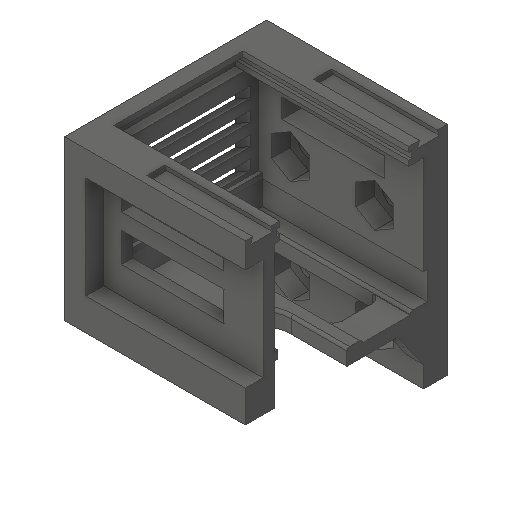
# Autodesk Inventor part: sensor-house-reflection
Saved by Autodesk Inventor 2022 (Build 260153000, 153)
## iProperties
Created: 2016-08-30
Part Number: sensor-house-reflection
Material: ABS Plastic
Document SubType Name: Modeling
Designer: Max
Density: 1.06 g/cm^3
Appearance: Gray
Mass: 12.7799 g
Surface Area: 104.372 cm^2
Volume: 12.0565 cm^3
Author: Max
Autodesk Inventor part; units mm, degrees
ref_plane "YZ Plane" through (0, 0, 0) normal (1, 0, 0) x (0, 1, 0)
ref_plane "XZ Plane" through (0, 0, 0) normal (0, 1, 0) x (-1, 0, 0)
ref_plane "XY Plane" through (0, 0, 0) normal (0, 0, 1) x (1, 0, 0)
sketch "Sketch1" plane through (0, 0, 0) normal (0, 1, 0) x (-1, 0, 0)
  line L0 (0, 0) -> (31.267, 0)
  line L1 (31.267, 0) -> (31.267, -29.05)
  line L2 (31.267, -29.05) -> (0, -29.05)
  line L3 (0, -29.05) -> (0, 0)
  line L4 (34.267, -32.05) -> (34.267, 3)
  line L5 (34.267, 3) -> (-3, 3)
  line L6 (-3, 3) -> (-3, -32.05)
  line L7 (-3, -32.05) -> (34.267, -32.05)
  line L8 (0, 3) -> (0, 0)
  line L9 (0, -29.05) -> (0, -32.05)
  dimension "d0" = 29.05
  dimension "d1" = 31.267
  dimension "d2" = 3
  constraints: 20 end point, 4 parallel, 3 point on line, 2 perpendicular, 1 horizontal, 1 vertical, 3 other
  measures "d0" distance of L0.end L1.end
  measures "d1" distance of L1.end L2.end
  measures "d2" distance between parallel lines of L1 L4
extrude "Extrusion1" add sketch "Sketch1" along normal blind 6.26 contours L8 L5 L4 L7 L9 L2 L1 L0
sketch "Sketch2" plane through (0, 6.26, 0) normal (0, 1, 0) x (1, 0, 0)
  line L0 (0, 0) -> (-31.267, 0) construction
  line L1 (-31.267, 0) -> (-31.267, 29.05) construction
  line L2 (-31.267, 29.05) -> (0, 29.05) construction
  line L3 (0, 29.05) -> (0, 32.05) construction
  line L4 (0, 32.05) -> (-34.267, 32.05) construction
  line L5 (-34.267, 32.05) -> (-34.267, -3) construction
  line L6 (-34.267, -3) -> (0, -3) construction
  line L7 (0, -3) -> (0, 0) construction
  line L8 (-34.267, 32.05) -> (-34.267, -3) projected
  line L9 (0, -3) -> (0, 0) projected
  line L10 (-34.267, -3) -> (0, -3)
  line L11 (0, -3) -> (0, 0.7)
  line L12 (0, 0.7) -> (-30.567, 0.7)
  line L13 (0, 0) -> (-31.267, 0) construction
  line L14 (-30.567, 0.7) -> (-30.567, 28.35)
  line L15 (-31.267, 0) -> (-31.267, 29.05) construction
  line L16 (-30.567, 28.35) -> (0, 28.35)
  line L17 (0, 29.05) -> (0, 32.05) projected
  line L18 (0, 28.35) -> (0, 32.05)
  line L19 (0, 32.05) -> (-34.267, 32.05) projected
  line L20 (0, 32.05) -> (-34.267, 32.05)
  line L21 (-34.267, 32.05) -> (-34.267, -3)
  dimension "d5" = 0.7
  dimension "d6" = 0.7
  dimension "d7" = 0.7
  constraints: 16 end point, 4 perpendicular, 2 parallel, 1 collinear, 1 horizontal, 1 point on line
  measures "d5" distance between parallel lines of L0 L12
  measures "d6" distance between parallel lines of L1 L14
  measures "d7" distance between parallel lines of L2 L16
extrude "Extrusion2" add sketch "Sketch2" against normal blind 1
sketch "Sketch3" plane through (0, 5.26, 0) normal (0, -1, 0) x (1, 0, 0)
  line L0 (-31.267, 0) -> (0, 0) construction
  line L1 (-31.267, -29.05) -> (-31.267, 0) construction
  line L2 (0, -29.05) -> (-31.267, -29.05) construction
  line L3 (0, -29.05) -> (0, -28.35) construction
  line L4 (0, -28.35) -> (-30.567, -28.35) construction
  line L5 (-30.567, -28.35) -> (-30.567, -0.7) construction
  line L6 (-30.567, -0.7) -> (0, -0.7) construction
  line L7 (0, -0.7) -> (0, 0) construction
  line L8 (0, -0.7) -> (0, 0) projected
  line L9 (0, 0) -> (-31.267, 0) projected
  line L10 (0, -0.7) -> (-30.567, -0.7)
  line L11 (-30.567, -0.7) -> (-30.567, 0)
  line L12 (-30.567, 0) -> (0, 0)
  line L13 (0, 0) -> (0, -0.7)
  constraints: 8 end point, 2 parallel, 1 collinear, 1 horizontal, 1 perpendicular, 1 point on line
extrude "Extrusion3" add sketch "Sketch3" along normal blind 0.5
sketch "Sketch4" plane through (0, 0, 0) normal (0, -1, 0) x (1, 0, 0)
  line L0 (0, 0) -> (-31.267, 0) projected
  line L1 (0, 3) -> (0, 0) projected
  line L2 (-34.267, 3) -> (0, 3) projected
  line L3 (-34.267, -32.05) -> (-34.267, 3) projected
  line L4 (0, -32.05) -> (-34.267, -32.05) projected
  line L5 (0, -29.05) -> (0, -32.05) projected
  line L6 (-31.267, -29.05) -> (0, -29.05) projected
  line L7 (-31.267, 0) -> (-31.267, -29.05) projected
extrude "Extrusion4" add sketch "Sketch4" against normal blind 24
sketch "Sketch7" plane through (0, 24, 0) normal (0, 1, 0) x (1, 0, 0)
  line L0 (0, 0.7) -> (-30.567, 0.7) construction
  line L1 (-30.567, 0.7) -> (-30.567, 28.35) construction
  line L2 (-30.567, 28.35) -> (0, 28.35) construction
  line L3 (-32.952, 1.015) -> (0, 1.015)
  line L4 (-32.952, 1.015) -> (-32.952, 25.535)
  line L5 (-32.952, 25.535) -> (0, 25.535)
  line L6 (0, -18.4949) -> (0, 56.6124) construction
  line L7 (-34.267, -3) -> (0, -3) projected
  line L8 (0, 1.015) -> (0, -3)
  line L9 (0, -3) -> (-34.267, -3)
  line L10 (-34.267, 32.05) -> (-34.267, -3) projected
  line L11 (-34.267, -3) -> (-34.267, 32.05)
  line L12 (-34.267, 32.05) -> (0, 32.05)
  line L13 (0, 29.05) -> (0, 32.05) projected
  line L14 (0, 25.535) -> (0, 32.05)
  point P0 (0, 0)
  dimension "d15" = 2.385
  dimension "d17" = 2.815
  dimension "d58" = 0.315
  constraints: 18 end point, 3 point on line, 3 vertical, 2 collinear, 2 horizontal, 2 perpendicular
  measures "d15" distance between parallel lines of L1 L4
  measures "d17" distance between parallel lines of L2 L5
  measures "d58" distance between parallel lines of L0 L3
extrude "Extrusion5" add sketch "Sketch7" along normal blind 1
sketch "Sketch8" plane through (0, 25, 0) normal (0, 1, 0) x (1, 0, 0)
  line L0 (0, 1.015) -> (-32.952, 1.015) construction
  line L1 (-32.952, 1.015) -> (-32.952, 25.535) construction
  line L2 (-32.952, 25.535) -> (0, 25.535) construction
  line L3 (0, 25.535) -> (0, 32.05) construction
  line L4 (0, 32.05) -> (-34.267, 32.05) construction
  line L5 (-34.267, 32.05) -> (-34.267, -3) construction
  line L6 (-34.267, -3) -> (0, -3) construction
  line L7 (0, -3) -> (0, 1.015) construction
  line L8 (0, -3) -> (0, 1.015) projected
  line L9 (0, 0.44) -> (-33.452, 0.44)
  line L10 (-33.452, 0.44) -> (-33.452, 26.11)
  line L11 (-33.452, 26.11) -> (0, 26.11)
  line L12 (0, 25.535) -> (0, 29.05) projected
  line L13 (0, 29.05) -> (0, 32.05) projected
  line L14 (0, 32.05) -> (-34.267, 32.05)
  line L15 (-34.267, -3) -> (0, -3) projected
  line L16 (-34.267, 32.05) -> (-34.267, -3) projected
  line L17 (-34.267, -3) -> (-34.267, 32.05)
  line L18 (-34.267, -3) -> (0, -3)
  line L19 (0, -3) -> (0, 0.44)
  line L20 (0, 26.11) -> (0, 32.05)
  point P0 (0, 0)
  dimension "d20" = 0.575
  dimension "d21" = 0.5
  dimension "d22" = 0.575
  constraints: 16 end point, 3 collinear, 3 perpendicular, 2 point on line, 1 horizontal, 1 vertical
  measures "d20" distance between parallel lines of L0 L9
  measures "d21" distance between parallel lines of L1 L10
  measures "d22" distance between parallel lines of L2 L11
extrude "Extrusion6" add sketch "Sketch8" along normal blind 1.25
sketch "Sketch9" plane through (0, 26.25, 0) normal (0, 1, 0) x (1, 0, 0)
  line L0 (0, 32.05) -> (-34.267, 32.05) construction
  line L1 (-34.267, 32.05) -> (-34.267, -3) construction
  line L2 (-34.267, -3) -> (0, -3) construction
  line L3 (0, -3) -> (0, 0.44) construction
  line L4 (0, 0.44) -> (-33.452, 0.44) construction
  line L5 (-33.452, 0.44) -> (-33.452, 26.11) construction
  line L6 (-33.452, 26.11) -> (0, 26.11) construction
  line L7 (0, 26.11) -> (0, 32.05) construction
  line L8 (0, 1.015) -> (-32.952, 1.015) construction
  line L9 (-32.952, 25.535) -> (0, 25.535) construction
  line L10 (-34.267, 32.05) -> (-34.267, -3) projected
  line L11 (-34.267, -3) -> (0, -3) projected
  line L12 (-34.267, -3) -> (0, -3)
  line L13 (-31.452, 1.015) -> (0, 1.015)
  line L14 (0, -3) -> (0, 1.015)
  line L15 (-31.452, 1.015) -> (-31.452, 25.535)
  line L16 (-31.452, 25.535) -> (0, 25.535)
  line L17 (0, 25.535) -> (0, 29.05) projected
  line L18 (0, 29.05) -> (0, 32.05) projected
  line L19 (0, 25.535) -> (0, 32.05)
  line L20 (0, 32.05) -> (-34.267, 32.05)
  line L21 (-34.267, -3) -> (-34.267, 32.05)
  dimension "d25" = 2
  constraints: 16 end point, 4 collinear, 2 perpendicular, 2 vertical, 1 point on line
  measures "d25" distance between parallel lines of L5 L15
extrude "Extrusion7" add sketch "Sketch9" along normal blind 1
sketch "Sketch10" plane through (0, 0, 0) normal (0, -1, 0) x (1, 0, 0)
  line L0 (-34.267, -32.05) -> (-34.267, 3) projected
  line L1 (0, -32.05) -> (-34.267, -32.05) projected
  line L2 (-34.267, 3) -> (0, 3)
  line L3 (0, 3) -> (0, -32.05)
  line L4 (0, -32.05) -> (-34.267, -32.05)
  line L5 (-34.267, -32.05) -> (-34.267, 3)
  point P0 (0, 0)
  constraints: 8 end point, 2 parallel, 1 horizontal, 1 perpendicular
extrude "Extrusion8" add sketch "Sketch10" along normal blind 3
sketch "Sketch11" plane through (0, -3, 0) normal (0, -1, 0) x (1, 0, 0)
  line L0 (-7.172, -16.735) -> (-26.102, -16.735)
  line L1 (-27.762, -18.395) -> (-27.762, -24.145)
  line L2 (-26.102, -25.805) -> (-7.172, -25.805)
  line L3 (-5.512, -24.145) -> (-5.512, -18.395)
  arc A0 (-5.512, -18.395) -> (-7.172, -16.735) centre (-7.172, -18.395) ccw
  arc A1 (-7.172, -25.805) -> (-5.512, -24.145) centre (-7.172, -24.145) ccw
  arc A2 (-26.102, -16.735) -> (-27.762, -18.395) centre (-26.102, -18.395) ccw
  arc A3 (-27.762, -24.145) -> (-26.102, -25.805) centre (-26.102, -24.145) ccw
  circle A4 centre (-10.572, -6.975) radius 6.835
  line L4 (-31.267, -29.05) -> (0, -29.05) construction
  line L5 (-31.267, 0) -> (-31.267, -29.05) construction
  line L6 (0, 0) -> (-31.267, 0) construction
  point P0 (-5.512, -16.735)
  point P1 (-27.762, -16.735)
  point P2 (-5.512, -25.805)
  dimension "d30" = 9.07
  dimension "d31" = 22.25
  dimension "d32" = 1.66
  dimension "d33" = 13.67
  dimension "d34" = 3.245
  dimension "d35" = 3.505
  dimension "d36" = 20.695
  dimension "d37" = 6.975
  constraints: 8 end point, 8 point on circle, 8 tangent, 6 point on line, 5 centre point, 3 equal radius, 2 parallel, 1 horizontal, 1 perpendicular
  measures "d30" distance of point (-5.512, -25.805) point (-5.512, -16.735)
  measures "d31" distance of point (-5.512, -16.735) point (-27.762, -16.735)
  measures "d32" radius of A0
  measures "d33" diameter of A4
  measures "d34" distance between parallel lines of L4 L2
  measures "d35" distance between parallel lines of L5 L1
  measures "d36" distance from line of L5 A4.centre
  measures "d37" distance from line of L6 A4.centre
extrude "Extrusion9" cut sketch "Sketch11" against normal blind 3
sketch "Sketch12" plane through (0, 24, -25.535) normal (1, 0, 0) x (0, 0, -1)
  line L0 (0.27, -27) -> (0.27, -24) construction
  line L1 (0.27, -27) -> (0.27, -24) construction
  line L2 (-8.8, -27) -> (-8.8, -24) construction
  line L3 (-8.8, -27) -> (-8.8, -24) construction
  line L4 (-8.8, -24) -> (0.27, -24)
  line L5 (0.27, -24) -> (0.27, -24.6)
  line L6 (0.27, -24.6) -> (-8.8, -24.6)
  line L7 (-8.8, -24.6) -> (-8.8, -24)
  point P0 (-25.535, -24)
  dimension "d40" = 0.6
  constraints: 8 end point, 2 parallel, 1 horizontal, 1 perpendicular, 1 point on line
  measures "d40" distance between parallel lines of L6 L4
extrude "Extrusion10" cut sketch "Sketch12" against normal blind 10
sketch "Sketch13" plane through (0, 24, -25.535) normal (1, 0, 0) x (0, 0, -1)
  line L0 (-25.395, -24) -> (-11.725, -24) construction
  line L1 (-11.725, -27) -> (-25.395, -27) construction
  line L2 (-25.395, -24) -> (-11.725, -24) projected
  line L3 (-25.395, -24) -> (-11.725, -24)
  line L4 (-11.725, -24) -> (-11.725, -27)
  line L5 (-11.725, -27) -> (-25.395, -27)
  line L6 (-25.395, -27) -> (-25.395, -24)
  point P0 (-25.535, -24)
  constraints: 8 end point, 2 parallel, 1 horizontal, 1 perpendicular
extrude "Extrusion11" cut sketch "Sketch13" against normal up to surface round surface about axis through (-10.572, -3, -6.975) along (0, 1, 0) radius 6.835 far side no
fillet "Fillet1" radius 0.5 8 edges at (-27.2758, 0, -17.2212) (-27.762, 0, -21.27) (-27.2758, 0, -25.3188) (-13.051, 0, -25.805) (-13.051, 0, -16.735) (-5.286, 0, -13.81) (-5.286, 0, -0.14) (-17.407, 0, -6.975)
sketch "Sketch16" plane through (-34.267, 27.25, 3) normal (0, 0, 1) x (1, 0, 0)
  line L0 (0, -30.25) -> (0, 0) construction
  line L1 (34.267, -30.25) -> (0, -30.25) construction
  line L2 (34.267, -30.25) -> (34.267, 0) construction
  line L3 (0, 0) -> (34.267, 0) construction
  line L4 (-13.0029, -10.46) -> (34.267, -10.46) construction
  line L5 (0, -7.185) -> (34.267, -7.185) construction
  line L6 (7.4, -6.758) -> (7.4, -10.36)
  line L7 (26.8405, -6.758) -> (26.8405, -10.46)
  line L8 (7.4, -6.758) -> (26.8405, -6.758)
  line L9 (7.4, -10.36) -> (26.8405, -10.36)
  point P0 (34.267, -27.25)
  dimension "d59" = 19.79
  dimension "d65" = 3.602
  dimension "d66" = 19.4405
  dimension "d67" = 7.4
  dimension "d155" = 10.36
  constraints: 12 end point, 5 point on line, 3 parallel, 2 horizontal, 1 vertical
  measures "d59" distance between parallel lines of L1 L4
  measures "d65" distance between parallel lines of L9 L8
  measures "d66" distance of L6.start L7.start
  measures "d67" distance between parallel lines of L0 L6
  measures "d155" distance between parallel lines of L3 L9
extrude "Extrusion14" cut sketch "Sketch16" against normal through all
thicken "Thicken1" operation add thickness 2.475 both sides no extend neighbours yes toward (0, 0, 1) faces at (-13.8978, 3.63, 3)
sketch "available_for_screw" plane through (-31.267, 6.26, -29.05) normal (0, 0, 1) x (1, 0, 0)
  line L0 (-0.185, 20.99) -> (31.267, 20.99) construction
  line L1 (1, 9.79) -> (30.267, 9.79) construction
  line L2 (30.267, 9.79) -> (30.267, 0.1) construction
  line L3 (30.267, 0.1) -> (1, 0.1) construction
  line L4 (1, 0.1) -> (1, 9.79) construction
  line L5 (31.267, 0) -> (0, 0) construction
  line L6 (0, 0) -> (0, 17.74) construction
  line L7 (31.267, 0) -> (31.267, 17.74) construction
  point P0 (31.267, -6.26)
  dimension "d82" = 11.2
  dimension "d83" = 0.1
  dimension "d84" = 1
  dimension "d85" = 1
  constraints: 8 end point, 2 parallel, 1 horizontal, 1 perpendicular
  measures "d82" distance between parallel lines of L1 L0
  measures "d83" distance between parallel lines of L5 L3
  measures "d84" distance between parallel lines of L6 L4
  measures "d85" distance between parallel lines of L7 L2
thicken "Thicken2" operation add thickness 0.8 both sides no extend neighbours yes toward (0, 0, -1) faces at (-13.8978, 3.63, -32.05)
sketch "Sketch20" plane through (-31.267, 6.26, -29.05) normal (0, 0, 1) x (1, 0, 0)
  line L0 (6, 1.1793) -> (2.44, 3.2346)
  line L1 (2.44, 3.2346) -> (2.44, 7.3454)
  line L2 (2.44, 7.3454) -> (6, 9.4007)
  line L3 (6, 9.4007) -> (9.56, 7.3454)
  line L4 (9.56, 7.3454) -> (9.56, 3.2346)
  line L5 (9.56, 3.2346) -> (6, 1.1793)
  line L6 (0, 0) -> (0, 17.74) projected
  line L7 (1, 9.79) -> (30.267, 9.79) construction
  circle A0 centre (6, 5.29) radius 2.04
  line L8 (22, 1.1793) -> (18.44, 3.2346)
  line L9 (18.44, 3.2346) -> (18.44, 7.3454)
  line L10 (18.44, 7.3454) -> (22, 9.4007)
  line L11 (22, 9.4007) -> (25.56, 7.3454)
  line L12 (25.56, 7.3454) -> (25.56, 3.2346)
  line L13 (25.56, 3.2346) -> (22, 1.1793)
  line L14 (31.267, 0) -> (31.267, 17.74) projected
  circle A1 centre (22, 5.29) radius 2.04
  point P0 (31.267, -6.26)
  dimension "d88" = 6
  dimension "d89" = 7.12
  dimension "d90" = 4.5
  dimension "d91" = 4.08
  dimension "d92" = 7.12
  dimension "d94" = 16
  dimension "d95" = 4.08
  constraints: 24 end point, 2 centre point, 2 coincident, 2 vertical, 1 horizontal alignment, 26 other
  measures "d88" distance from line of L6 point (6, 5.29)
  measures "d89" distance between parallel lines of L4 L1
  measures "d90" distance from line of point (6, 5.29) L7
  measures "d91" diameter of A0
  measures "d92" distance between parallel lines of L12 L9
  measures "d94" distance of point (6, 5.29) point (22, 5.29)
  measures "d95" diameter of A1
extrude "Extrusion17" cut sketch "Sketch20" against normal through all contours A0 | A1
extrude "Extrusion18" cut sketch "Sketch20" against normal blind 2.8
thicken "Thicken4" operation add thickness 0.7 both sides no extend neighbours yes toward (0, 0, 1) faces at (-12.8978, 22.8307, -29.05)
sketch "Sketch21" plane through (0, -3, -32.85) normal (0, 0, -1) x (-1, 0, 0)
  line L0 (34.267, 0) -> (0, 0) construction
  line L1 (0, 0) -> (34.267, 0)
  line L2 (34.267, 0) -> (34.267, -11)
  line L3 (34.267, -11) -> (0, -11)
  line L4 (0, -11) -> (0, 0)
  line L5 (34.267, 0) -> (34.267, 30.25) construction
  circle A0 centre (9.267, -5.1107) radius 2.04
  circle A1 centre (9.267, 14.55) radius 2.04 construction
  circle A2 centre (9.267, 14.55) radius 2.04 construction
  line L6 (9.267, 10.4393) -> (12.827, 12.4946) construction
  line L7 (5.707, 12.4946) -> (9.267, 10.4393) construction
  line L8 (5.707, 16.6054) -> (5.707, 12.4946) construction
  line L9 (9.267, 18.6607) -> (5.707, 16.6054) construction
  line L10 (12.827, 16.6054) -> (9.267, 18.6607) construction
  line L11 (12.827, 12.4946) -> (12.827, 16.6054) construction
  circle A3 centre (25.267, 14.55) radius 2.04 construction
  line L12 (25.267, 10.4393) -> (28.827, 12.4946) construction
  line L13 (21.707, 12.4946) -> (25.267, 10.4393) construction
  line L14 (21.707, 16.6054) -> (21.707, 12.4946) construction
  line L15 (25.267, 18.6607) -> (21.707, 16.6054) construction
  line L16 (28.827, 16.6054) -> (25.267, 18.6607) construction
  line L17 (28.827, 12.4946) -> (28.827, 16.6054) construction
  line L18 (9.267, -9.2215) -> (5.707, -7.1661)
  line L19 (5.707, -7.1661) -> (5.707, -3.0554)
  line L20 (5.707, -3.0554) -> (9.267, -1)
  line L21 (9.267, -1) -> (12.827, -3.0554)
  line L22 (12.827, -3.0554) -> (12.827, -7.1661)
  line L23 (12.827, -7.1661) -> (9.267, -9.2215)
  circle A4 centre (25.267, -5.1107) radius 2.04
  line L24 (25.267, -9.2215) -> (21.707, -7.1661)
  line L25 (21.707, -7.1661) -> (21.707, -3.0554)
  line L26 (21.707, -3.0554) -> (25.267, -1)
  line L27 (25.267, -1) -> (28.827, -3.0554)
  line L28 (28.827, -3.0554) -> (28.827, -7.1661)
  line L29 (28.827, -7.1661) -> (25.267, -9.2215)
  point P0 (0, 3)
  dimension "d104" = 11
  dimension "d105" = 7.12
  dimension "d106" = 1
  dimension "d107" = 4.08
  dimension "d108" = 4.08
  dimension "d109" = 7.12
  constraints: 32 end point, 2 centre point, 2 coincident, 2 parallel, 2 vertical, 2 vertical alignment, 1 collinear, 1 horizontal, 1 horizontal alignment, 1 perpendicular, 26 other
  measures "d104" distance of L3.end L0.end
  measures "d105" distance between parallel lines of L22 L19
  measures "d106" distance from line of L0 L20.end
  measures "d107" diameter of A0
  measures "d108" diameter of A4
  measures "d109" distance between parallel lines of L28 L25
extrude "Extrusion19" add sketch "Sketch21" against normal up to surface (4.5 mm away) contours L1 L2 L3 L4 | L18 L19 L20 L21 L22 L23 | L24 L25 L26 L27 L28 L29
sketch "Sketch22" plane through (-34.267, -3, -28.35) normal (0, 0, 1) x (1, 0, 0)
  line L0 (25, -1) -> (21.44, -3.0554) projected
  line L1 (28.56, -3.0554) -> (25, -1) projected
  line L2 (28.56, -7.1661) -> (28.56, -3.0554) projected
  line L3 (25, -9.2215) -> (28.56, -7.1661) projected
  line L4 (21.44, -7.1661) -> (25, -9.2215) projected
  line L5 (21.44, -3.0554) -> (21.44, -7.1661) projected
  line L6 (12.56, -7.1661) -> (12.56, -3.0554) projected
  line L7 (9, -9.2215) -> (12.56, -7.1661) projected
  line L8 (5.44, -7.1661) -> (9, -9.2215) projected
  line L9 (5.44, -3.0554) -> (5.44, -7.1661) projected
  line L10 (9, -1) -> (5.44, -3.0554) projected
  line L11 (12.56, -3.0554) -> (9, -1) projected
  point P0 (34.267, 3)
extrude "Extrusion20" cut sketch "Sketch22" against normal blind 3.5
sketch "Sketch24" plane through (-34.267, -3, 5.475) normal (-1, 0, 0) x (0, 0, 1)
  line L0 (-33.825, -11) -> (-33.825, 0) construction
  line L1 (0, 0) -> (-33.825, 0) construction
  line L2 (-33.825, -7.1661) -> (-33.825, -3.0554) construction
  line L3 (-33.825, -7) -> (-28.825, 0)
  line L4 (-33.825, -7) -> (-33.825, 0)
  line L5 (-28.825, 0) -> (-33.825, 0)
  point P0 (-5.475, 3)
  dimension "d118" = 5
  constraints: 6 end point, 1 collinear, 1 point on line, 1 vertical
  measures "d118" distance from line of L0 L3.end
extrude "Extrusion21" add sketch "Sketch24" against normal blind 3
sketch "Sketch25" plane through (0, 25, -26.11) normal (1, 0, 0) x (0, 0, -1)
  line L0 (-2.76, -28) -> (2.24, -35) projected
  line L1 (2.24, -28) -> (2.24, -35) projected
  line L2 (-2.76, -28) -> (2.24, -28) projected
  point P0 (-26.11, -25)
extrude "Extrusion22" add sketch "Sketch25" against normal blind 3
sketch "Sketch26" plane through (-34.267, -3, 5.475) normal (-1, 0, 0) x (0, 0, 1)
  line L0 (-32.325, 22.25) -> (-6, 22.25)
  line L1 (-6, 22.25) -> (-6, 20.25)
  line L2 (-6, 20.25) -> (-32.325, 20.25)
  line L3 (-32.325, 20.25) -> (-32.325, 22.25)
  line L4 (-33.825, -7) -> (-28.825, 0) construction
  line L5 (0, 0) -> (-28.825, 0) construction
  line L6 (0, 0) -> (0, 30.25) construction
  line L7 (-38.325, 30.25) -> (0, 30.25) construction
  line L8 (-38.325, -11) -> (-38.325, 30.25) construction
  line L9 (-33.825, 19.89) -> (-33.825, 23.492) construction
  line L10 (-33.825, 23.492) -> (-33.825, 19.89) construction
  line L11 (-33.825, 12.4946) -> (-33.825, 10.4393) construction
  line L12 (-33.825, 10.4393) -> (-33.825, 12.4946) construction
  line L13 (-33.825, 12.4946) -> (-33.825, 16.6054) construction
  line L14 (-33.825, 16.6054) -> (-33.825, 18.6607) construction
  line L15 (-33.825, 18.6607) -> (-33.825, 16.6054) construction
  line L16 (-33.825, 16.6054) -> (-33.825, 12.4946) construction
  line L17 (-33.825, 12.4946) -> (-33.825, 10.4393) construction
  line L18 (-33.825, 10.4393) -> (-33.825, 12.4946) construction
  line L19 (-33.825, 12.4946) -> (-33.825, 16.6054) construction
  line L20 (-33.825, 16.6054) -> (-33.825, 18.6607) construction
  line L21 (-33.825, 18.6607) -> (-33.825, 16.6054) construction
  line L22 (-33.825, 16.6054) -> (-33.825, 12.4946) construction
  line L23 (-33.825, 9.26) -> (-33.825, 8.26) construction
  line L24 (-33.825, 8.26) -> (-33.825, 27) construction
  line L25 (-33.825, 9.26) -> (-33.825, 27) construction
  line L26 (-32.325, 16.25) -> (-32.325, 18.25)
  line L27 (-6, 16.25) -> (-32.325, 16.25)
  line L28 (-32.325, 18.25) -> (-6, 18.25)
  line L29 (-6, 18.25) -> (-6, 16.25)
  line L30 (-32.325, 12.25) -> (-32.325, 14.25)
  line L31 (-6, 12.25) -> (-32.325, 12.25)
  line L32 (-32.325, 14.25) -> (-6, 14.25)
  line L33 (-6, 14.25) -> (-6, 12.25)
  line L34 (-32.325, 8.25) -> (-32.325, 10.25)
  line L35 (-6, 8.25) -> (-32.325, 8.25)
  line L36 (-32.325, 10.25) -> (-6, 10.25)
  line L37 (-6, 10.25) -> (-6, 8.25)
  line L38 (-38.325, -11) -> (-33.825, -11) projected
  line L39 (-33.825, -11) -> (-33.825, -7) projected
  point P0 (-5.475, 3)
  dimension "d124" = 8
  dimension "d125" = 2
  dimension "d126" = 6
  dimension "d127" = 6
  dimension "d130" = 4
  constraints: 32 end point, 2 parallel, 1 horizontal, 1 perpendicular, 1 vertical, 24 other
  measures "d124" distance between parallel lines of L7 L0
  measures "d125" distance of L2.end L0.start
  measures "d126" distance between parallel lines of L8 L3
  measures "d127" distance between parallel lines of L6 L1
  measures "d130" distance of L0.start L26.end
sketch "Sketch27" plane through (-34.267, -3, 5.475) normal (0, 0, 1) x (1, 0, 0)
  line L0 (34.267, 30.25) -> (0, 30.25) construction
  line L1 (0, 30.25) -> (4, 32.5594)
  point P0 (34.267, 3)
  dimension "d135" = 30
  dimension "d136" = 4
  constraints: 2 end point
  measures "d135" angle of L0 L1
  measures "d136" horizontal distance of L0.end L1.end
sweep "Sweep1" cut profiles "Sketch26" path "Sketch27"
sketch "Sketch28" plane through (-34.267, -3, 5.475) normal (0, 0, 1) x (1, 0, 0)
  line L0 (26.8405, 19.89) -> (7.4, 19.89) construction
  line L1 (7.4, 19.89) -> (7.4, 23.492) construction
  line L2 (7.4, 23.492) -> (26.8405, 23.492) construction
  line L3 (26.8405, 23.492) -> (26.8405, 19.89) construction
  line L4 (0, 0) -> (0, 30.25) construction
  line L5 (34.267, 0) -> (0, 0) construction
  line L6 (34.267, 0) -> (34.267, 30.25) construction
  line L7 (0, 30.25) -> (34.267, 30.25) construction
  line L8 (4, 25.492) -> (34.267, 25.492)
  line L9 (34.267, 25.492) -> (34.267, 6.0515)
  line L10 (34.267, 6.0515) -> (4, 6.0515)
  line L11 (4, 6.0515) -> (4, 25.492)
  line L12 (0, 0) -> (0, 30.25) construction
  point P0 (34.267, 3)
  dimension "d139" = 4
  dimension "d140" = 19.4405
  dimension "d141" = 2
  constraints: 8 end point, 2 parallel, 1 horizontal, 1 perpendicular, 1 point on line
  measures "d139" distance between parallel lines of L11 L12
  measures "d140" distance between parallel lines of L10 L8
  measures "d141" distance between parallel lines of L2 L8
extrude "Extrusion23" cut sketch "Sketch28" against normal blind 3.375
chamfer "Chamfer2" distance 4 angle 45 1 edges at (-34.267, -14, -30.6)
sketch "Sketch29" plane through (-34.267, -3, 2.1) normal (0, 0, 1) x (1, 0, 0)
  line L0 (26.8405, 23.492) -> (7.4, 23.492) construction
  line L1 (26.8405, 19.89) -> (26.8405, 23.492) construction
  line L2 (7.4, 19.89) -> (26.8405, 19.89) construction
  line L3 (7.4, 23.492) -> (7.4, 19.89) construction
  line L4 (4, 25.492) -> (34.267, 25.492) construction
  line L5 (4, 6.0515) -> (4, 25.492) construction
  line L6 (34.267, 6.0515) -> (4, 6.0515) construction
  line L7 (34.267, 25.492) -> (34.267, 6.0515) construction
  line L8 (7.4, 16.89) -> (26.8405, 16.89)
  line L9 (26.8405, 16.89) -> (26.8405, 11.26)
  line L10 (26.8405, 11.26) -> (7.4, 11.26)
  line L11 (7.4, 11.26) -> (7.4, 16.89)
  line L12 (3, 9.26) -> (34.267, 9.26) construction
  point P0 (34.267, 3)
  dimension "d147" = 3
  dimension "d151" = 2
  constraints: 8 end point, 2 collinear, 2 parallel, 1 horizontal, 1 perpendicular
  measures "d147" distance between parallel lines of L8 L2
  measures "d151" distance between parallel lines of L12 L10
extrude "Extrusion24" cut sketch "Sketch29" against normal blind 10
sketch "Sketch30" plane through (-34.267, -3, 2.1) normal (0, 0, 1) x (1, 0, 0)
  line L0 (26.8405, 23.492) -> (7.4, 23.492) construction
  line L1 (7.4, 23.492) -> (7.4, 19.89) projected
  line L2 (7.4, 23.492) -> (26.8405, 23.492)
  line L3 (26.8405, 23.492) -> (26.8405, 23.592)
  line L4 (26.8405, 23.592) -> (7.4, 23.592)
  line L5 (7.4, 23.592) -> (7.4, 23.492)
  line L6 (26.8405, 19.89) -> (26.8405, 23.492) projected
  point P0 (34.267, 3)
  dimension "d152" = 0.1
  constraints: 8 end point, 2 parallel, 1 collinear, 1 horizontal, 1 perpendicular
  measures "d152" distance between parallel lines of L0 L4
ref_plane "Work Plane1" through (-46.167, -14, -32.95) normal (0, 0, 1) x (1, 0, 0)
extrude "Extrusion25" cut sketch "Sketch30" against normal up to surface (35.05 mm away)
sketch "Sketch45" plane through (0, 4.76, -0.7) normal (1, 0, 0) x (0, 0, -1)
  line L0 (-6.175, 17.732) -> (-2.8, 17.732) projected
  line L1 (-2.8, 17.732) -> (-2.8, -1.7085) projected
  line L2 (-2.8, -1.7085) -> (-6.175, -1.7085) projected
  line L3 (-6.175, -7.76) -> (-6.175, -1.7085) projected
  line L4 (-0.56, -7.76) -> (-6.175, -7.76) projected
  line L5 (-0.56, -7.76) -> (-0.56, -5.26) projected
  arc A0 (-0.56, -5.26) -> (-0.7, -4.913) centre (-1.06, -5.26) ccw projected
  line L6 (-0.7, 0) -> (-0.7, -4.913) projected
  line L7 (0, 0) -> (-0.7, 0) projected
  line L8 (0, 1.5) -> (0, 0) projected
  line L9 (-0.7, 1.5) -> (0, 1.5) projected
  line L10 (-0.7, 1.5) -> (-0.7, 19.24) projected
  line L11 (-0.7, 19.24) -> (0.315, 19.24) projected
  line L12 (0.315, 19.24) -> (0.315, 20.24) projected
  line L13 (-0.26, 20.24) -> (0.315, 20.24) projected
  line L14 (-0.26, 20.24) -> (-0.26, 21.49) projected
  line L15 (-0.26, 21.49) -> (0.315, 21.49) projected
  line L16 (0.315, 21.49) -> (0.315, 22.49) projected
  line L17 (-6.175, 22.49) -> (0.315, 22.49) projected
  line L18 (-6.175, 17.732) -> (-6.175, 22.49) projected
  line L19 (27.65, 0.5) -> (27.65, 19.24) projected
  line L20 (28.35, 0.5) -> (27.65, 0.5) projected
  line L21 (28.35, -4.76) -> (28.35, 0.5) projected
  line L22 (28.35, -4.76) -> (25.605, -4.76) projected
  arc A1 (25.605, -4.76) -> (25.105, -5.26) centre (25.605, -5.26) ccw projected
  line L23 (25.105, -5.26) -> (25.105, -5.36) projected
  line L24 (25.105, -5.36) -> (16.035, -5.36) projected
  line L25 (16.035, -5.36) -> (16.035, -5.26) projected
  arc A2 (16.035, -5.26) -> (15.535, -4.76) centre (15.535, -5.26) ccw projected
  line L26 (15.535, -4.76) -> (13.61, -4.76) projected
  arc A3 (13.61, -4.76) -> (13.11, -5.26) centre (13.61, -5.26) ccw projected
  line L27 (13.11, -5.26) -> (13.11, -7.76) projected
  line L28 (22.65, -7.76) -> (13.11, -7.76) projected
  line L29 (22.65, -7.76) -> (27.65, -14.76) projected
  line L30 (27.65, -14.76) -> (27.65, -18.76) projected
  line L31 (32.15, -18.76) -> (27.65, -18.76) projected
  line L32 (32.15, -18.76) -> (32.15, 22.49) projected
  line L33 (24.835, 22.49) -> (32.15, 22.49) projected
  line L34 (24.835, 21.49) -> (24.835, 22.49) projected
  line L35 (24.835, 21.49) -> (25.41, 21.49) projected
  line L36 (25.41, 20.24) -> (25.41, 21.49) projected
  line L37 (24.835, 20.24) -> (25.41, 20.24) projected
  line L38 (24.835, 19.24) -> (24.835, 20.24) projected
  line L39 (24.835, 19.24) -> (27.65, 19.24) projected
  line L40 (-6.175, 22.49) -> (0.315, 22.49) projected
  line L41 (-4.7746, 22.49) -> (-5.175, 21.39)
  line L42 (-5.175, 21.39) -> (-0.975, 21.39)
  line L43 (-0.975, 21.39) -> (-1.3754, 22.49)
  line L44 (24.835, 22.49) -> (32.15, 22.49) projected
  line L45 (26.8504, 22.49) -> (26.45, 21.39)
  line L46 (26.45, 21.39) -> (30.65, 21.39)
  line L47 (30.65, 21.39) -> (30.2496, 22.49)
  point P0 (-0.7, -4.76)
  dimension "d243" = 1.1
  dimension "d244" = 70
  dimension "d245" = 70
  dimension "d246" = 4.2
  dimension "d247" = 1
  dimension "d248" = 4.2
  dimension "d249" = 1.5
  dimension "d250" = 70
  dimension "d251" = 70
  dimension "d252" = 1.1
  constraints: 12 end point, 4 point on line, 2 parallel
  measures "d243" distance between parallel lines of L17 L42
  measures "d244" angle of L42 L43
  measures "d245" angle of L42 L41
  measures "d246" distance of L41.end L42.end
  measures "d247" distance from line of L18 L41.end
  measures "d248" distance of L45.end L46.end
  measures "d249" distance from line of L32 L46.end
  measures "d250" angle of L46 L47
  measures "d251" angle of L46 L45
  measures "d252" distance between parallel lines of L46 L33
extrude "Extrusion43" cut sketch "Sketch45" against normal blind 20.1 contours L17 L43 L42 L41 | L33 L47 L46 L45
sketch "Sketch31" plane through (0, 27.25, 0) normal (0, 1, 0) x (1, 0, 0)
  line L0 (0, 32.85) -> (-34.267, 32.85) projected
  line L1 (-34.267, 32.85) -> (-34.267, -5.475) projected
  line L2 (-34.267, -5.475) -> (0, -5.475) projected
  line L3 (0, -5.475) -> (0, 1.015) projected
  line L4 (0, 1.015) -> (-31.452, 1.015) projected
  line L5 (-31.452, 1.015) -> (-31.452, 25.535) projected
  line L6 (-31.452, 25.535) -> (0, 25.535) projected
  line L7 (0, 25.535) -> (0, 32.85) projected
  line L8 (-30.267, 32.85) -> (0, 32.85) projected
  line L9 (-25.612, 32.85) -> (-13.512, 32.85)
  line L10 (-13.512, 32.85) -> (-13.512, -5.475)
  line L11 (-13.512, -5.475) -> (-25.612, -5.475)
  line L12 (-25.612, -5.475) -> (-25.612, 32.85)
  point P0 (0, 0)
  dimension "d166" = 12.1
  dimension "d196" = 5.84
  constraints: 8 end point, 2 parallel, 2 point on line, 1 horizontal, 1 perpendicular
  measures "d166" distance between parallel lines of L10 L12
  measures "d196" distance between parallel lines of L5 L12
sketch "Sketch32" plane through (0, 28.75, 0) normal (0, 1, 0) x (1, 0, 0)
  line L0 (-25.612, 7.995) -> (-13.512, 7.995)
  line L1 (-13.512, 7.995) -> (-13.512, 9.995)
  line L2 (-13.512, 20.195) -> (-25.612, 20.195)
  line L3 (-25.612, 20.195) -> (-25.612, 18.195)
  line L4 (-25.612, 32.85) -> (-25.612, -5.475) projected
  line L5 (-13.512, -5.475) -> (-13.512, 32.85) projected
  line L6 (-24.612, 19.195) -> (-14.512, 19.195)
  line L7 (-14.512, 19.195) -> (-14.512, 18.195)
  line L8 (-14.512, 8.995) -> (-24.612, 8.995)
  line L9 (-24.612, 8.995) -> (-24.612, 9.995)
  line L10 (-24.612, 18.195) -> (-25.612, 18.195)
  line L11 (-14.512, 18.195) -> (-13.512, 18.195)
  line L12 (-24.612, 9.995) -> (-25.612, 9.995)
  line L13 (-25.612, 25.535) -> (-25.612, 1.015) projected
  line L14 (-14.512, 9.995) -> (-13.512, 9.995)
  line L15 (-13.512, 32.85) -> (-25.612, 32.85) projected
  line L16 (-24.612, 18.195) -> (-24.612, 19.195)
  line L17 (-25.612, 18.195) -> (-25.612, 9.995)
  line L18 (-24.612, 9.995) -> (-24.612, 18.195)
  line L19 (-25.612, 9.995) -> (-25.612, 7.995)
  line L20 (-14.512, 9.995) -> (-14.512, 8.995)
  line L21 (-13.512, 9.995) -> (-13.512, 18.195)
  line L22 (-14.512, 18.195) -> (-14.512, 9.995)
  line L23 (-13.512, 18.195) -> (-13.512, 20.195)
  line L24 (-13.512, 25.535) -> (0, 25.535) projected
  point P0 (0, 0)
  dimension "d158" = 10.2
  dimension "d159" = 10.1
  dimension "d161" = 1
  dimension "d162" = 1
  dimension "d163" = 1
  dimension "d167" = 1
  dimension "d168" = 1
  dimension "d169" = 1
  dimension "d170" = 1
  dimension "d194" = 6.34
  constraints: 40 end point, 20 parallel, 10 perpendicular, 7 collinear, 4 point on line, 3 horizontal
  measures "d158" distance of L6.end L8.start
  measures "d159" distance of L8.start L8.end
  measures "d161" distance between parallel lines of L0 L8
  measures "d162" distance from line of L2 L6.start
  measures "d163" distance between parallel lines of L1 L7
  measures "d167" distance between parallel lines of L6 L10
  measures "d168" distance between parallel lines of L6 L11
  measures "d169" distance between parallel lines of L8 L14
  measures "d170" distance between parallel lines of L8 L12
  measures "d194" distance between parallel lines of L6 L24
sketch "Sketch39" plane through (0, 27.25, 0) normal (0, -1, 0) x (1, 0, 0)
  line L0 (-13.512, -1.015) -> (-25.612, -1.015) projected
  line L1 (-25.612, -25.535) -> (-25.612, -1.015) projected
  line L2 (-25.612, -25.535) -> (-13.512, -25.535) projected
  line L3 (-13.512, -1.015) -> (-13.512, -25.535) projected
  line L4 (-13.512, -7.995) -> (-25.612, -7.995) projected
  line L5 (-25.612, -20.195) -> (-13.512, -20.195) projected
  point P0 (0, 0)
sketch "Sketch40" plane through (0, 28.75, 0) normal (0, 1, 0) x (1, 0, 0)
  line L0 (-24.612, 9.995) -> (-24.612, 8.995) projected
  line L1 (-14.512, 18.195) -> (-14.512, 19.195) projected
  line L2 (-24.612, 8.995) -> (-14.512, 8.995)
  line L3 (-14.512, 8.995) -> (-14.512, 19.195)
  line L4 (-14.512, 19.195) -> (-24.612, 19.195)
  line L5 (-24.612, 19.195) -> (-24.612, 8.995)
  point P0 (0, 0)
  constraints: 8 end point, 2 parallel, 1 horizontal, 1 perpendicular
sketch "Sketch41" plane through (0, 27.55, 0) normal (0, 1, 0) x (1, 0, 0)
  line L0 (-24.112, 9.495) -> (-15.012, 9.495)
  line L1 (-15.012, 9.495) -> (-15.012, 18.695)
  line L2 (-15.012, 18.695) -> (-24.112, 18.695)
  line L3 (-24.112, 18.695) -> (-24.112, 9.495)
  line L4 (-14.512, 8.995) -> (-24.612, 8.995) projected
  line L5 (-14.512, 19.195) -> (-14.512, 8.995) projected
  line L6 (-24.612, 19.195) -> (-14.512, 19.195) projected
  line L7 (-24.612, 8.995) -> (-24.612, 19.195) projected
  point P0 (0, 0)
  dimension "d202" = 0.5
  dimension "d203" = 0.5
  dimension "d204" = 0.5
  dimension "d205" = 0.5
  dimension "d238" = 45
  dimension "d239" = 0.5
  constraints: 10 end point, 4 point on circle, 4 tangent, 2 centre point, 2 equal length, 1 midpoint, 1 point on line
  measures "d238" angle of L0 L7
sketch "Sketch43" plane through (-13.512, 27.25, -25.535) normal (1, 0, 0) x (0, 0, -1)
  line L0 (-6.34, 0.3) -> (-16.54, 0.3) projected
  line L1 (-16.54, 9.5) -> (-16.54, 0.3) projected
  line L2 (-6.34, 9.5) -> (-6.34, 0.3) projected
  line L3 (0, 0.5) -> (0, 0) projected
  line L4 (7.315, 0) -> (0, 0) projected
  line L5 (7.315, 0) -> (7.315, 1.5) projected
  line L6 (-5.34, 1.5) -> (7.315, 1.5) projected
  line L7 (-5.34, 1.5) -> (-5.34, 9.5) projected
  line L8 (-7.34, 9.5) -> (-5.34, 9.5) projected
  line L9 (-7.34, 1.5) -> (-7.34, 9.5) projected
  line L10 (-15.54, 1.5) -> (-7.34, 1.5) projected
  line L11 (-15.54, 1.5) -> (-15.54, 9.5) projected
  line L12 (-17.54, 9.5) -> (-15.54, 9.5) projected
  line L13 (-17.54, 1.5) -> (-17.54, 9.5) projected
  line L14 (-31.01, 1.5) -> (-17.54, 1.5) projected
  line L15 (-31.01, 0) -> (-31.01, 1.5) projected
  line L16 (-24.52, 0) -> (-31.01, 0) projected
  line L17 (-24.52, 0) -> (-24.52, 0.5) projected
  line L18 (-24.52, 0.5) -> (-17.54, 0.5) projected
  line L19 (-17.54, 0.5) -> (-17.54, 0) projected
  line L20 (-17.54, 0) -> (-5.34, 0) projected
  line L21 (-5.34, 0) -> (-5.34, 0.5) projected
  line L22 (-5.34, 0.5) -> (0, 0.5) projected
  line L23 (-24.52, 0.5) -> (-17.54, 0.5) projected
  line L24 (-17.54, 0.5) -> (-16.04, 0.5)
  line L25 (-5.64, 9.3232) -> (-5.64, 0.1232) projected
  line L26 (-17.54, 0) -> (-5.34, 0) projected
  line L27 (-16.04, 0.3) -> (-16.04, 0) projected
  line L28 (-6.84, 0.3) -> (-6.84, 0) projected
  line L29 (-15.54, 1.5) -> (-16.54, 1.5)
  line L30 (-7.34, 1.5) -> (-6.34, 1.5)
  line L31 (-16.04, 0.3) -> (-16.04, 0.5)
  line L32 (-6.84, 0.3) -> (-6.84, 0.5)
  line L33 (-16.04, 0.5) -> (-6.84, 0.5)
  line L34 (-16.04, 0.5) -> (-16.04, 1.5)
  line L35 (-6.84, 0.5) -> (-6.84, 1.5)
  line L36 (-6.84, 0.5) -> (-5.34, 0.5)
  point P0 (-25.535, -27.25)
  point P1 (-16.54, 0.5)
  point P2 (-6.34, 0.5)
  constraints: 18 end point, 9 point on line, 4 perpendicular, 2 midpoint
sketch "Sketch44" plane through (-25.612, 28.75, -7.995) normal (0, 0, 1) x (1, 0, 0)
  line L0 (1, -1.2) -> (11.1, -1.2) projected
  line L1 (1, -1.2) -> (10.2, 8)
  line L2 (1, -1.2) -> (10.2, 8) construction
  line L3 (0.8232, -1.0232) -> (10.0232, 8.1768)
  line L4 (10.3768, 7.8232) -> (1.1768, -1.3768)
  arc A0 (0.8232, -1.0232) -> (1.1768, -1.3768) centre (1, -1.2) ccw
  arc A1 (10.3768, 7.8232) -> (10.0232, 8.1768) centre (10.2, 8) ccw
  line L5 (0, 8) -> (12.1, 8) projected
  point P0 (25.612, -28.75)
  point P1 (5.6, 3.4)
  dimension "d234" = 45
  dimension "d235" = 0.5
  constraints: 10 end point, 4 point on circle, 4 tangent, 2 centre point, 1 midpoint, 1 parallel, 1 point on line
  measures "d234" angle of L0 L1
  measures "d235" distance between parallel lines of L4 L3
sketch "Sketch34" plane through (0, 27.75, 0) normal (0, 1, 0) x (1, 0, 0)
  line L0 (-13.512, 9.995) -> (-14.512, 9.995) projected
  line L1 (-13.512, 18.195) -> (-13.512, 9.995) projected
  line L2 (-14.512, 18.195) -> (-13.512, 18.195) projected
  line L3 (-14.512, 19.195) -> (-14.512, 18.195) projected
  line L4 (-24.612, 19.195) -> (-14.512, 19.195) projected
  line L5 (-24.612, 18.195) -> (-24.612, 19.195) projected
  line L6 (-25.612, 18.195) -> (-24.612, 18.195) projected
  line L7 (-25.612, 9.995) -> (-25.612, 18.195) projected
  line L8 (-24.612, 9.995) -> (-25.612, 9.995) projected
  line L9 (-24.612, 8.995) -> (-24.612, 9.995) projected
  line L10 (-14.512, 8.995) -> (-24.612, 8.995) projected
  line L11 (-14.512, 9.995) -> (-14.512, 8.995) projected
  line L12 (-24.312, 9.295) -> (-14.812, 9.295)
  line L13 (-14.812, 9.295) -> (-14.812, 18.895)
  line L14 (-14.812, 18.895) -> (-24.312, 18.895)
  line L15 (-24.312, 18.895) -> (-24.312, 9.295)
  point P0 (0, 0)
  dimension "d178" = 0.3
  dimension "d179" = 0.3
  dimension "d180" = 0.3
  dimension "d181" = 0.3
  constraints: 8 end point, 2 parallel, 1 horizontal, 1 perpendicular
  measures "d178" distance between parallel lines of L10 L12
  measures "d179" distance between parallel lines of L4 L14
  measures "d180" distance between parallel lines of L3 L13
  measures "d181" distance between parallel lines of L5 L15
sketch "Sketch35" plane through (0, 27.75, 0) normal (0, 1, 0) x (1, 0, 0)
  line L0 (-14.812, 18.895) -> (-14.812, 9.295) projected
  line L1 (-14.812, 9.295) -> (-24.312, 9.295) projected
  line L2 (-24.312, 9.295) -> (-24.312, 18.895) projected
  line L3 (-24.312, 18.895) -> (-14.812, 18.895) projected
  line L4 (-13.512, 9.995) -> (-14.512, 9.995) projected
  line L5 (-13.512, 18.195) -> (-13.512, 9.995) projected
  line L6 (-14.512, 18.195) -> (-13.512, 18.195) projected
  line L7 (-14.512, 19.195) -> (-14.512, 18.195) projected
  line L8 (-24.612, 19.195) -> (-14.512, 19.195) projected
  line L9 (-24.612, 18.195) -> (-24.612, 19.195) projected
  line L10 (-25.612, 18.195) -> (-24.612, 18.195) projected
  line L11 (-25.612, 9.995) -> (-25.612, 18.195) projected
  line L12 (-24.612, 9.995) -> (-25.612, 9.995) projected
  line L13 (-24.612, 8.995) -> (-24.612, 9.995) projected
  line L14 (-14.512, 8.995) -> (-24.612, 8.995) projected
  line L15 (-14.512, 9.995) -> (-14.512, 8.995) projected
  line L16 (-24.612, 8.995) -> (-24.612, 9.995) projected
  line L17 (-24.612, 9.995) -> (-24.612, 18.195)
  line L18 (-14.512, 19.195) -> (-14.512, 18.195) projected
  line L19 (-14.512, 9.995) -> (-14.512, 18.195)
  point P0 (0, 0)
  constraints: 4 end point, 2 collinear
sketch "Sketch37" plane through (-25.612, 28.25, -7.995) normal (0, 0, 1) x (1, 0, 0)
  line L0 (1.3, -0.5) -> (10.8, -0.5) projected
  line L1 (12.1, 0) -> (0, 0) projected
  line L2 (12.1, 0) -> (12.1, 8) projected
  line L3 (0, 8) -> (12.1, 8) projected
  line L4 (0, 0) -> (0, 8) projected
  line L5 (10.8, -0.5) -> (2.3, 8)
  line L6 (11.1, 8) -> (1, 8) projected
  line L7 (2.3, 8) -> (10.8, -0.5) construction
  line L8 (2.1232, 7.8232) -> (10.6232, -0.6768)
  line L9 (10.9768, -0.3232) -> (2.4768, 8.1768)
  arc A0 (2.4768, 8.1768) -> (2.1232, 7.8232) centre (2.3, 8) ccw
  arc A1 (10.6232, -0.6768) -> (10.9768, -0.3232) centre (10.8, -0.5) ccw
  point P0 (25.612, -28.25)
  point P1 (6.55, 3.75)
  dimension "d190" = 45
  dimension "d191" = 0.5
  constraints: 10 end point, 4 point on circle, 4 tangent, 2 centre point, 1 midpoint, 1 parallel, 1 point on line
  measures "d190" angle of L0 L5
  measures "d191" distance between parallel lines of L8 L9
sketch "Sketch36" plane through (-13.512, 28.25, -20.195) normal (0, 0, -1) x (-1, 0, 0)
  line L0 (11.1, 0) -> (11.1, 8) projected
  line L1 (1, 0) -> (1, 8) projected
  line L2 (12.1, 0) -> (0, 0) projected
  line L3 (12.1, 0) -> (12.1, 8) projected
  line L4 (0, 8) -> (12.1, 8) projected
  line L5 (0, 0) -> (0, 8) projected
  line L6 (0, 0) -> (12.1, 0) projected
  line L7 (-6.0855, -11.36) -> (-6.0855, -7.658) projected
  line L8 (-6.0855, -7.658) -> (13.355, -7.658) projected
  line L9 (13.355, -7.658) -> (13.355, -11.36) projected
  line L10 (13.355, -11.36) -> (-6.0855, -11.36) projected
  circle A0 centre (-4.245, -16.7) radius 2.04 projected
  circle A1 centre (11.755, -16.7) radius 2.04 projected
  circle A2 centre (-4.245, -36.3607) radius 2.04 projected
  circle A3 centre (11.755, -36.3607) radius 2.04 projected
  line L11 (20.755, -38.25) -> (16.755, -42.25) projected
  line L12 (20.755, -38.25) -> (20.755, -1) projected
  line L13 (12.1, -1) -> (20.755, -1) projected
  line L14 (12.1, -1) -> (12.1, 0) projected
  line L15 (0, 0) -> (12.1, 0) projected
  line L16 (0, -1) -> (0, 0) projected
  line L17 (-13.512, -1) -> (0, -1) projected
  line L18 (-13.512, -42.25) -> (-13.512, -1) projected
  line L19 (16.755, -42.25) -> (-13.512, -42.25) projected
  line L20 (11.1, -0.5) -> (1, -0.5) projected
  line L21 (-6.0855, -7.658) -> (13.355, -7.658) projected
  line L22 (12.1, -1) -> (0, -1) projected
  line L23 (1, -0.5) -> (9.5, 8)
  line L24 (1, -0.5) -> (9.5, 8) construction
  line L25 (0.8232, -0.3232) -> (9.3232, 8.1768)
  line L26 (9.6768, 7.8232) -> (1.1768, -0.6768)
  arc A4 (0.8232, -0.3232) -> (1.1768, -0.6768) centre (1, -0.5) ccw
  arc A5 (9.6768, 7.8232) -> (9.3232, 8.1768) centre (9.5, 8) ccw
  point P0 (-13.512, -28.25)
  point P1 (5.25, 3.75)
  dimension "d186" = 45
  dimension "d187" = 0.5
  constraints: 10 end point, 4 point on circle, 4 tangent, 2 centre point, 2 equal length, 1 midpoint, 1 point on line
  measures "d186" angle of L20 L23
  measures "d187" distance between parallel lines of L26 L25
body "Solid1"
